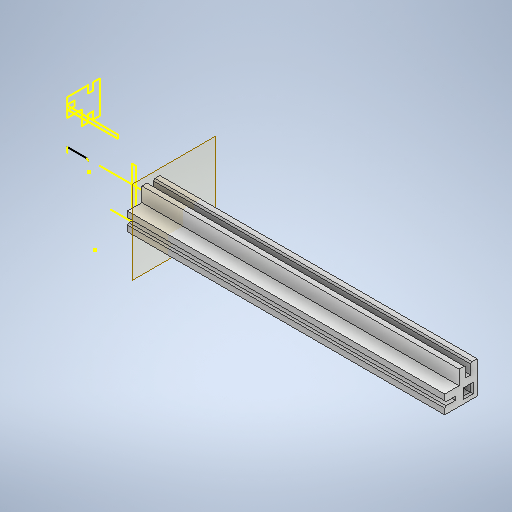
# Autodesk Inventor part: Kątownik_219mm_pleaxe_na około x3szt
Saved by Autodesk Inventor 2025 (Build 290162000, 162)
## iProperties
Created: 2025-07-30
Part Number: Kątownik_219mm_pleaxe_na około x3szt
Material: Ogólny
Document SubType Name: Modeling
Designer: ThePi
Density: 1 g/cm^3
Appearance: Domyślna
Author: ThePi
Autodesk Inventor part; units mm, degrees
ref_plane "YZ Plane" through (0, 0, 0) normal (1, 0, 0) x (0, 1, 0)
ref_plane "XZ Plane" through (0, 0, 0) normal (0, 1, 0) x (-1, 0, 0)
ref_plane "XY Plane" through (0, 0, 0) normal (0, 0, 1) x (1, 0, 0)
sketch "Szkic1" plane through (0, 0, 0) normal (1, 0, 0) x (0, 1, 0)
  line L0 (0, 0) -> (0, 22.5)
  line L1 (0, 0) -> (22.5, 0)
  line L2 (22.5, 12.5) -> (12.5, 12.5)
  line L3 (12.5, 22.5) -> (12.5, 12.5)
  line L4 (4.5, 22.5) -> (4.5, 17.5)
  line L5 (22.5, 8) -> (17.5, 8)
  line L6 (22.5, 8) -> (22.5, 12.5)
  line L7 (8, 17.5) -> (8, 22.5)
  line L8 (8, 22.5) -> (12.5, 22.5)
  line L9 (4.5, 22.5) -> (0, 22.5)
  line L10 (22.5, 12.5) -> (22.5, 8)
  line L11 (22.5, 8) -> (17.5, 8)
  line L12 (17.5, 4.5) -> (22.5, 4.5)
  line L13 (22.5, 4.5) -> (22.5, 0)
  line L14 (4.5, 17.5) -> (4.5, 15)
  line L15 (4.5, 15) -> (8, 15)
  line L16 (8, 15) -> (8, 17.5)
  line L17 (17.5, 8) -> (15, 8)
  line L18 (15, 8) -> (15, 4.5)
  line L19 (15, 4.5) -> (17.5, 4.5)
  dimension "d0" = 22.5
  dimension "d7" = 22.5
  dimension "d41" = 3.5
  dimension "d48" = 2.5
  dimension "d49" = 3.5
  dimension "d50" = 2.5
  dimension "d51" = 3.5
  constraints: 40 end point, 4 perpendicular, 3 horizontal, 3 vertical, 2 collinear
  measures "d0" distance of L0.start L0.end
  measures "d7" distance of L0.start L1.end
  measures "d41" distance of L5.end L12.start
  measures "d48" distance of L4.end L14.end
  measures "d49" distance of L14.end L15.end
  measures "d50" distance of L5.end L17.end
  measures "d51" distance of L17.end L18.end
extrude "Wyciągnięcie proste1" add sketch "Szkic1" along normal blind 220
sketch "Szkic2" plane through (220, 0, 0) normal (1, 0, 0) x (0, 0, -1)
  line L0 (-12.5, 22.5) -> (-12.5, 12.5) projected
  line L1 (-12.5, 12.5) -> (-12.5, 0)
  line L2 (-22.5, 0) -> (0, 0) projected
  line L3 (-12.5, 0) -> (0, 0)
  line L4 (0, 0) -> (0, 12.5)
  line L5 (-12.5, 12.5) -> (-22.5, 12.5) projected
  line L6 (0, 12.5) -> (-12.5, 12.5)
  line L7 (-8.75, 6.25) -> (-8.75, 8.75)
  line L8 (-8.75, 8.75) -> (-3.75, 8.75)
  line L9 (-3.75, 8.75) -> (-3.75, 3.75)
  line L10 (-3.75, 3.75) -> (-8.75, 3.75)
  line L11 (-8.75, 3.75) -> (-8.75, 8.75)
  constraints: 18 end point, 5 perpendicular, 2 point on line, 1 collinear, 1 vertical
extrude "Wyciągnięcie proste3" cut sketch "Szkic2" against normal blind 17 contours L7 L8 L9 L10 L11
sketch "Szkic3" plane through (0, 0, 0) normal (-1, 0, 0) x (0, 0, 1)
  line L0 (12.5, 12.5) -> (22.5, 12.5) projected
  line L1 (12.5, 12.5) -> (12.5, 0)
  line L2 (22.5, 0) -> (0, 0) projected
  line L3 (12.5, 0) -> (0, 0)
  line L4 (0, 0) -> (0, 12.5)
  line L5 (0, 12.5) -> (12.5, 12.5)
  line L6 (8.75, 8.75) -> (3.75, 8.75) projected
  line L7 (6.25, 8.75) -> (8.75, 8.75)
  line L8 (8.75, 8.75) -> (8.75, 3.75)
  line L9 (8.75, 3.75) -> (3.75, 3.75)
  line L10 (3.75, 3.75) -> (3.75, 8.75)
  line L11 (3.75, 8.75) -> (8.75, 8.75)
  constraints: 18 end point, 5 perpendicular, 1 horizontal, 1 point on line, 1 vertical
extrude "Wyciągnięcie proste4" cut sketch "Szkic3" against normal blind 17 contours L8 L9 L10 L6
chamfer "Faza5" distance 1 angle 45 8 edges at (0, 3.75, 6.25) (0, 6.25, 8.75) (0, 8.75, 6.25) (0, 6.25, 3.75) (220, 8.75, 6.25) (220, 6.25, 3.75) (220, 6.25, 8.75) (220, 3.75, 6.25)
sketch "Szkic4" plane through (0, 0, 0) normal (0, -1, 0) x (1, 0, 0)
  point P0 (0, 0)
thicken "Pogrubienie2" operation add thickness 0.5 both sides no extend neighbours no toward (0, 1, 0) faces at (146.6667, 4.5, 17.5)
thicken "Pogrubienie3" operation add thickness 0.5 both sides no extend neighbours no toward (0, -1, 0) faces at (146.6667, 8, 20)
chamfer "Faza7" distance 1 angle 45 4 edges at (110, 22.5, 4.5) (110, 22.5, 8) (110, 7.5, 22.5) (110, 5, 22.5)
derived "Narożnik Środek LEWY Plexa.ipt"
feature "Bryła1::Narożnik Środek LEWY Plexa.ipt" [suppressed]
sketch "Szkic3_1" plane through (0, 0, 0) normal (0, -1, 0) x (1, 0, 0)
  point P0 (0, 0)
ref_plane "Płaszczyzna konstrukcyjna1" through (28.25, 0, 15) normal (1, 0, 0) x (0, 0, -1)
sketch "Szkic18" plane through (-19.25, 52.5, 45) normal (0, 0, 1) x (1, 0, 0)
  line L0 (0, -3.5) -> (0, 0) projected
  line L1 (14.5, -1) -> (13.5, 0) projected
  line L2 (0, 0) -> (13.5, 0)
  line L3 (13.5, 0) -> (14.5, -1)
  point P0 (19.25, -52.5)
  constraints: 4 end point, 1 collinear, 1 horizontal
sketch "Szkic8" plane through (-49.25, 0, -7.5) normal (-1, 0, 0) x (0, 0, 1)
  point P0 (7.5, 0)
sketch "Szkic9" plane through (0, 0, 0) normal (0, -1, 0) x (1, 0, 0)
  point P0 (0, 0)
sketch "Szkic11" plane through (0, 0, 0) normal (0, -1, 0) x (1, 0, 0)
  point P0 (0, 0)
sketch "Szkic15" plane through (-1.75, 0, 15) normal (0, 0, 1) x (1, 0, 0)
  line L0 (0, 0) -> (0, 30) projected
  line L1 (0, 0) -> (0, 35) projected
  line L2 (0, 35) -> (0, 0) projected
  line L3 (-2.5, 0) -> (-2.5, 30) projected
  line L4 (0, 0) -> (-2.5, 0) projected
  line L5 (5, 0) -> (-17.5, 0) projected
  line L6 (-2.5, 0) -> (-2.5, 35) projected
  line L7 (-2.5, 35) -> (0, 35) projected
  line L8 (0, 0) -> (0, 35) projected
  line L9 (-17.5, 45) -> (-47.5, 45) projected
  line L10 (-47.5, 45) -> (-12.5, 45) projected
  line L11 (-12.5, 45) -> (-47.5, 45) projected
  line L12 (-47.5, 47.5) -> (-17.5, 47.5) projected
  line L13 (-47.5, 45) -> (-47.5, 47.5) projected
  line L14 (-47.5, 47.5) -> (-12.5, 47.5) projected
  line L15 (-12.5, 47.5) -> (-12.5, 45) projected
  point P0 (1.75, 0)
sketch "Szkic22" plane through (-9.25, 0, 45) normal (0, 0, 1) x (1, 0, 0)
  point P0 (9.25, 0)
sketch "Szkic32" plane through (0, 0, 0) normal (0, -1, 0) x (1, 0, 0)
  line L0 (-49.25, -7.5) -> (3.25, -7.5) projected
  line L1 (3.25, -7.5) -> (-0.5, -7.5) projected
  line L2 (-0.5, -7.5) -> (-4.25, -7.5) projected
  line L3 (-4.25, -7.5) -> (-0.5, -7.5) projected
  line L4 (-0.5, -7.5) -> (-0.5, -3.75) projected
  line L5 (-0.5, -3.75) -> (-5.5, -3.75) projected
  line L6 (-5.5, -3.75) -> (-5.5, 1.25) projected
  line L7 (-5.5, 1.25) -> (-0.5, 1.25) projected
  line L8 (-0.5, 1.25) -> (-0.5, -3.75) projected
  point P0 (0, 0)
sketch "Szkic33" plane through (-49.25, 0, -7.5) normal (-1, 0, 0) x (0, 0, 1)
  line L0 (4.5, 30) -> (4.5, 35) projected
  line L1 (4.5, 35) -> (8, 35) projected
  line L2 (8, 35) -> (8, 30) projected
  line L3 (8, 30) -> (12.5, 30) projected
  line L4 (12.5, 30) -> (12.5, 40) projected
  line L5 (12.5, 40) -> (22.5, 40) projected
  line L6 (22.5, 44.5) -> (22.5, 40) projected
  line L7 (22.5, 44.5) -> (17.5, 44.5) projected
  line L8 (17.5, 44.5) -> (17.5, 48) projected
  line L9 (17.5, 48) -> (22.5, 48) projected
  line L10 (22.5, 52.5) -> (22.5, 48) projected
  line L11 (4.5, 52.5) -> (0, 52.5) projected
  line L12 (8, 52.5) -> (8, 47.5) projected
  line L13 (8, 47.5) -> (4.5, 47.5) projected
  line L14 (4.5, 47.5) -> (4.5, 52.5) projected
  line L15 (22.5, 52.5) -> (8, 52.5) projected
  line L16 (0, 52.5) -> (0, 30) projected
  line L17 (0, 30) -> (4.5, 30) projected
  point P0 (7.5, 0)
